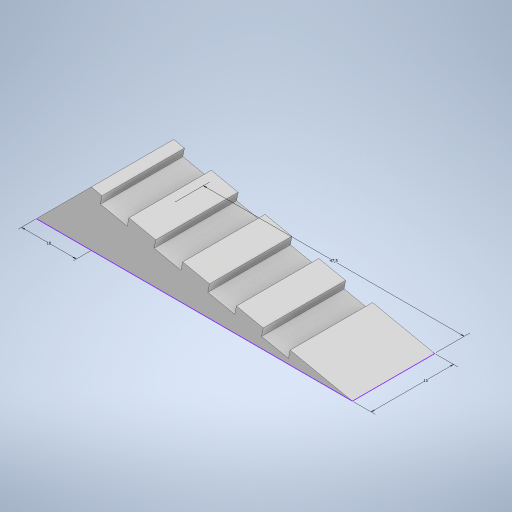
# Autodesk Inventor part: Keilvertsell
Saved by Autodesk Inventor 2023.1 (Build 271208000, 208)
## iProperties
Created: 2022-09-24
Part Number: Keilvertsell
Material: Generisch
Document SubType Name: Modeling
Designer: schwa
Density: 1 g/cm^3
Appearance: Vorgabe
Author: schwa
Autodesk Inventor part; units mm, degrees
ref_plane "YZ Plane" through (0, 0, 0) normal (1, 0, 0) x (0, 1, 0)
ref_plane "XZ Plane" through (0, 0, 0) normal (0, 1, 0) x (-1, 0, 0)
ref_plane "XY Plane" through (0, 0, 0) normal (0, 0, 1) x (1, 0, 0)
sketch "Skizze1" plane through (0, 0, 0) normal (0, 1, 0) x (-1, 0, 0)
  line L0 (18.599, 2.8535) -> (-28.901, 2.8535)
  line L1 (-28.901, 2.8535) -> (-28.901, -12.1465)
  line L2 (-28.901, -12.1465) -> (18.599, -12.1465)
  line L3 (18.599, -12.1465) -> (18.599, 2.8535)
  line L4 (18.599, -12.1465) -> (28.599, -12.1465)
  line L5 (28.599, -12.1465) -> (28.599, 2.8535)
  line L6 (28.599, 2.8535) -> (18.599, 2.8535)
  line L7 (18.599, 2.8535) -> (18.599, -12.1465)
  point P0 (0, 0)
  dimension "d0" = 47.5
  dimension "d1" = 15
  dimension "d6" = 10
  constraints: 16 end point, 4 parallel, 2 horizontal, 2 perpendicular
  measures "d0" distance of L2.end L1.end
  measures "d1" distance between parallel lines of L2 L0
  measures "d6" distance of L6.end L5.end
extrude "Extrusion1" add sketch "Skizze1" along normal blind 10 contours L3 L2 L1 L0
sketch "Skizze2" plane through (-18.599, 0, 2.8535) normal (0, 0, 1) x (1, 0, 0)
  line L0 (47.5, 10) -> (0, 10) projected
  line L1 (47.5, 0) -> (0, 10)
  line L2 (0, 10) -> (47.5, 10)
  line L3 (47.5, 10) -> (47.5, 0)
  point P0 (18.599, 0)
  constraints: 6 end point, 1 perpendicular
extrude "Extrusion2" cut sketch "Skizze2" against normal up to surface (15 mm away)
sketch "Skizze3" plane through (28.901, 0, 2.8535) normal (0.206, 0.9785, 0) x (0.9785, -0.206, 0)
  point P0 (-28.2811, 2.8535)
extrude "Extrusion3" add sketch "Skizze1" along normal blind 10 contours L6 L5 L4 L3
sketch "Skizze6" plane through (-28.599, 0, 2.8535) normal (0, 0, 1) x (1, 0, 0)
  line L0 (10, 10) -> (0, 10) projected
  line L1 (0, 0) -> (0, 10) projected
  line L2 (10, 10) -> (0, 0)
  line L3 (0, 0) -> (0, 10)
  line L4 (57.5, 0) -> (10, 10) projected
  line L5 (0, 10) -> (10, 10)
  point P0 (28.599, 0)
  constraints: 6 end point, 1 collinear, 1 perpendicular
extrude "Extrusion4" cut sketch "Skizze6" against normal blind 15
sketch "Skizze7" plane through (28.901, 0, 2.8535) normal (0.206, 0.9785, 0) x (0.9785, -0.206, 0)
  line L0 (0, 15) -> (-56.2666, 15) projected
  line L1 (-56.2666, 0) -> (0, 0) projected
  line L2 (-46.5412, 15) -> (-41.5412, 15)
  line L3 (-41.5412, 15) -> (-41.5412, 0)
  line L4 (-41.5412, 0) -> (-46.5412, 0)
  line L5 (-46.5412, 0) -> (-46.5412, 15)
  line L6 (-48.5412, 15) -> (-48.5412, 0) projected
  line L7 (-31.5412, 15) -> (-31.5412, 0)
  line L8 (-36.5412, 15) -> (-31.5412, 15)
  line L9 (-36.5412, 0) -> (-36.5412, 15)
  line L10 (-31.5412, 0) -> (-36.5412, 0)
  line L11 (-21.5412, 15) -> (-21.5412, 0)
  line L12 (-26.5412, 15) -> (-21.5412, 15)
  line L13 (-26.5412, 0) -> (-26.5412, 15)
  line L14 (-21.5412, 0) -> (-26.5412, 0)
  line L15 (-11.5412, 15) -> (-11.5412, 0)
  line L16 (-16.5412, 15) -> (-11.5412, 15)
  line L17 (-16.5412, 0) -> (-16.5412, 15)
  line L18 (-11.5412, 0) -> (-16.5412, 0)
  point P0 (-28.2811, 2.8535)
  point P1 (-16.5412, 15)
  point P2 (-16.5412, 0)
  point P3 (-11.5412, 0)
  point P4 (-11.5412, 15)
  point P5 (-26.5412, 0)
  point P6 (-21.5412, 0)
  point P7 (-21.5412, 15)
  point P8 (-36.5412, 0)
  point P9 (-31.5412, 0)
  point P10 (-31.5412, 15)
  point P11 (-46.5412, 0)
  point P12 (-41.5412, 15)
  dimension "d11" = 5
  dimension "d12" = 2
  dimension "d15" = 10
  constraints: 32 end point, 2 horizontal, 2 parallel, 2 point on line, 1 perpendicular, 24 other
  measures "d11" distance of L3.end L4.end
  measures "d12" distance between parallel lines of L6 L5
  measures "d15" distance of L2.end L7.start
extrude "Extrusion5" cut sketch "Skizze7" against normal blind 1.5 contours L15 L1 L17 L0 | L11 L1 L13 L0 | L7 L1 L9 L0 | L3 L1 L5 L0
